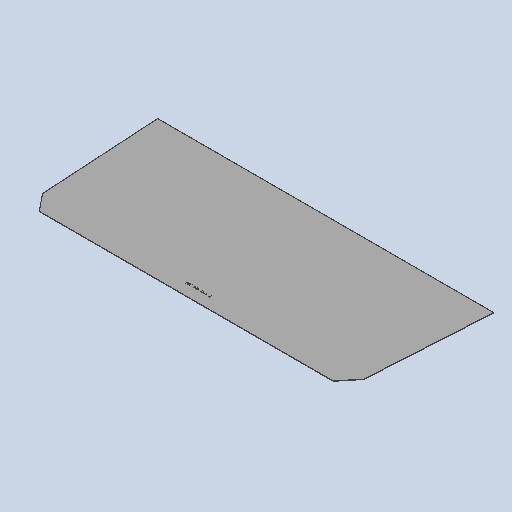
# Autodesk Inventor part: MSC 075 face 2
Saved by Autodesk Inventor 2025 (Build 290162010, 162A)
## iProperties
Created: 2024-06-16
Part Number: MSC 075 face 2
Material: AISI304
Document SubType Name: Sheet Metal
Designer: admin
Density: 8 g/cm^3
Sheet Metal Rule: AISI304 2mm Die16
Appearance: Default
Stock Number: МОО 075 морда 2
Flat Pattern Width: 66.1867 cm
Flat Pattern Length: 159.495 cm
Flat Pattern Area: 10556.4 cm^2
Sheet Metal Width: 661,867 mm
Sheet Metal Length: 1594,950 mm
Sheet Metal Area: 1055644,858 mm^2
Author: admin
Autodesk Inventor part; units mm, degrees
ref_plane "YZ Plane" through (0, 0, 0) normal (1, 0, 0) x (0, 1, 0)
ref_plane "XZ Plane" through (0, 0, 0) normal (0, 1, 0) x (-1, 0, 0)
ref_plane "XY Plane" through (0, 0, 0) normal (0, 0, 1) x (1, 0, 0)
sketch "Sketch1" plane through (0, 0, 0) normal (0, 0, 1) x (1, 0, 0)
  line L0 (797.4752, 0) -> (797.4752, -661.8669) construction
  line L1 (797.4752, -661.8669) -> (0, -661.8669)
  line L2 (751.1573, -579.8638) -> (684.3931, -661.8669) construction
  ellipse E0 centre (-10250, 795.2799) end of major axis (-10250.7907, -13633.3868) minor radius 11053 (753.0187, -574.9033) -> (782.4805, -83.0791) ccw construction
  line L3 (797.4752, 0) -> (762.6352, -581.6047)
  line L4 (697.2883, -661.8669) -> (797.4752, -538.8126)
  line L5 (753.0187, -574.9033) -> (763.0008, -575.5013) construction
  line L6 (782.4805, -83.0791) -> (792.4626, -83.6771) construction
  line L7 (0, -661.8669) -> (0, 0)
  line L8 (0, 0) -> (797.4752, 0)
  dimension "d3" = 10
  dimension "d4" = 10
  dimension "d5" = 10
  measures "d3" distance between parallel lines of L4 L2
  measures "d4" distance of L5.start L5.end
  measures "d5" distance of L6.start L6.end
extrude "Plate1" add sketch "Sketch1" along normal blind 2
mirror "Mirror1" about plane through (0, 0, 0) normal (1, 0, 0) of "Plate1"
sketch "Sketch2" plane through (0, 0, 2) normal (0, 0, 1) x (1, 0, 0)
  line L0 (-55, -611.8669) -> (-55, -599.8669) construction
  line L1 (-55, -599.8669) -> (55, -599.8669) construction
  line L2 (55, -599.8669) -> (55, -611.8669) construction
  line L3 (55, -611.8669) -> (-55, -611.8669) construction
  line L4 (-697.2883, -661.8669) -> (697.2883, -661.8669) projected
  point P0 (0, 0)
  point P1 (0, -611.8669)
  point P2 (0, -661.8669)
  dimension "d6" = 12
  dimension "d7" = 110
  dimension "d8" = 50
  constraints: 2 midpoint, 1 parallel, 1 vertical alignment, 2 other
  measures "d6" distance of L1.end L2.end
  measures "d7" distance between parallel lines of L0 L2
  measures "d8" distance between parallel lines of L4 L3
mark "Mark1"
equation "\"d2\" = Thickness"
equation "\"BendReliefWidth\" = Thickness"
equation "\"BendReliefDepth\" = 0.5 * Thickness"
equation "\"CornerReliefSize\" = 4 * Thickness"
equation "\"MinimumRemnant\" = 2 * Thickness"
equation "\"TransitionRadius\" = BendRadius"
equation "\"JacobiRadiusSize\" = BendRadius"
equation "\"GapSize\" = Thickness"
equation "\"Thickness\" = 2"
equation "\"BendRadius\" = 2.75"
body "Solid1"
